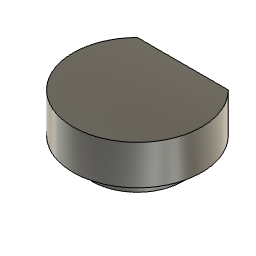
Kabeldruchführung (Autodesk Fusion 360 design; units mm, degrees)
Autodesk Fusion 360 part; units mm, degrees
note: some values were not read from the file. Set by a fixed rule: which sketch regions a step uses.
sketch "Sketch1" plane through (0, 0, 0) normal (0, 0, 1) x (1, 0, 0)
  circle A0 centre (0, 0) radius 26.5
  circle A1 centre (0, 0) radius 37.5
  line L0 (-35.6931, 26.5) -> (64.3069, 26.5)
  line L1 (64.3069, 26.5) -> (64.3069, 11.5)
  line L2 (64.3069, 11.5) -> (-35.6931, 11.5)
  line L3 (-35.6931, 11.5) -> (-35.6931, 26.5)
  line L4 (-35.6931, 26.5) -> (64.3069, 26.5)
  line L5 (64.3069, 26.5) -> (64.3069, 56.5)
  line L6 (64.3069, 56.5) -> (-35.6931, 56.5)
  line L7 (-35.6931, 56.5) -> (-35.6931, 26.5)
  circle A2 centre (0, 0) radius 20.5
  line L8 (-23.8747, 11.5) -> (-23.8747, 56.5)
  line L9 (23.8747, 11.5) -> (23.8747, 56.5)
  line L10 (18.4691, 8.8962) -> (23.8747, 11.5)
  line L11 (-23.8747, 11.5) -> (-18.4691, 8.8962)
  dimension "d1" = 53
  dimension "d2" = 75
  dimension "d3" = 100
  dimension "d4" = 15
  dimension "d5" = 30
  dimension "d12" = 41
  constraint coincident A0.centre A1.centre
  constraint horizontal L0
  constraint vertical L1
  constraint horizontal L2
  constraint vertical L3
  constraint tangent A0 L0
  constraint coincident A1 L2.end
  constraint horizontal L4
  constraint vertical L5
  constraint horizontal L6
  constraint vertical L7
  constraint collinear L1 L5
  constraint coincident A0 L8.start
  constraint coincident L2 L8.start
  constraint coincident L6 L8.end
  constraint perpendicular L6 L8
  constraint coincident A0 L9.start
  constraint coincident L2 L9.start
  constraint coincident L6 L9.end
  constraint perpendicular L6 L9
  constraint coincident A2 L10.start
  constraint coincident A2 L11.end
  constraint coincident A0.centre L11
  constraint coincident A0.centre L10
  measures "d1" diameter of A0
  measures "d2" diameter of A1
  measures "d3" distance of L0.start L0.end
  measures "d4" distance of L0.start L2.end
  measures "d5" distance of L0.start L6.end
  measures "d12" diameter of A2
extrude "Extrude1" add sketch "Sketch1" along normal blind 17 contours A0 A2 L10 L11 | A0 A1 L2 | A1 L0 L2 L4 L9 | A1 L0 L2 L4 L8
extrude "Extrude2" add sketch "Sketch1" along normal blind 6 from surface at 17 contours A0 A2 L10 L11 | A0 A1 L2 | A0 L2 A2 | A1 L0 L2 L4 L9 | L2 A2 L10 | A0 L0 L4 L9 | A0 L0 L4 L8 | A1 L0 L2 L4 L8 | L2 A2 L11 | L2 A2 | L2 A2
extrude "Extrude3" add sketch "Sketch1" against normal blind 10 contours A0 A2 L10 L11
equation "d2 = 53 mm + ( 2 * 11 ) * 1 mm"
equation "d12 = 53 mm - 12 mm"
